Autodesk Fusion 360 part; units mm, degrees
(part 2 of 2)
  spline S180 degree 3 poles (38.6443, -77.9749) (38.4375, -77.8397) (37.9935, -77.5493) (37.4619, -77.524) (37.1779, -77.5104) knots 0 0 0 0 0.0728 0.156317 0.156317 0.156317 0.156317
  spline S181 degree 3 poles (37.1779, -77.5104) (36.8852, -77.5181) (36.3595, -77.5319) (35.9103, -77.8002) (35.7111, -77.9191) knots 0 0 0 0 0.086047 0.154532 0.154532 0.154532 0.154532
  spline S182 degree 3 poles (35.7111, -77.9191) (35.5659, -78.0588) (35.2884, -78.3257) (35.2372, -78.7061) (35.2128, -78.8875) knots 0 0 0 0 0.058494 0.11181 0.11181 0.11181 0.11181
  spline S183 degree 3 poles (35.2128, -78.8875) (35.2207, -79.0001) (35.236, -79.2199) (35.3624, -79.4) (35.424, -79.4879) knots 0 0 0 0 0.033166 0.064726 0.064726 0.064726 0.064726
  spline S184 degree 3 poles (35.424, -79.4879) (35.5146, -79.5723) (35.7243, -79.7676) (35.9938, -79.8678) (36.1469, -79.9247) knots 0 0 0 0 0.036813 0.085194 0.085194 0.085194 0.085194
  spline S185 degree 3 poles (36.1469, -79.9247) (36.3404, -79.9828) (36.8751, -80.1434) (37.4173, -80.2768) (37.7633, -80.3619) knots 0 0 0 0 0.060601 0.167477 0.167477 0.167477 0.167477
  spline S186 degree 3 poles (37.7633, -80.3619) (38.237, -80.4825) (39.0523, -80.6899) (39.7493, -81.1565) (40.0412, -81.352) knots 0 0 0 0 0.14523 0.24996 0.24996 0.24996 0.24996
  spline S187 degree 3 poles (40.0412, -81.352) (40.3097, -81.6399) (40.8404, -82.2091) (40.9213, -82.9825) (40.9613, -83.3646) knots 0 0 0 0 0.1147 0.226743 0.226743 0.226743 0.226743
  spline S188 degree 3 poles (40.9613, -83.3646) (40.9427, -83.6159) (40.9051, -84.1229) (40.6564, -84.5664) (40.531, -84.7901) knots 0 0 0 0 0.074618 0.150525 0.150525 0.150525 0.150525
  spline S189 degree 3 poles (40.531, -84.7901) (40.3663, -85.001) (40.0277, -85.4343) (39.5352, -85.6799) (39.2822, -85.806) knots 0 0 0 0 0.07921 0.162795 0.162795 0.162795 0.162795
  spline S190 degree 3 poles (39.2822, -85.806) (38.9841, -85.9072) (38.3455, -86.124) (37.6706, -86.1429) (37.3108, -86.153) knots 0 0 0 0 0.093909 0.201185 0.201185 0.201185 0.201185
  spline S191 degree 3 poles (37.3108, -86.153) (36.7447, -86.1362) (35.7243, -86.1059) (34.8636, -85.5666) (34.4803, -85.3265) knots 0 0 0 0 0.16619 0.299601 0.299601 0.299601 0.299601
  spline S192 degree 3 poles (34.4803, -85.3265) (34.1997, -85.0227) (33.6242, -84.3996) (33.5278, -83.5554) (33.4784, -83.1228) knots 0 0 0 0 0.120771 0.247752 0.247752 0.247752 0.247752
  line L111 (33.4784, -83.1228) -> (35.4976, -83.035)
  spline S193 degree 3 poles (35.4976, -83.035) (35.5448, -83.2666) (35.6308, -83.6881) (35.9243, -83.9998) (36.0565, -84.1402) knots 0 0 0 0 0.069259 0.12604 0.12604 0.12604 0.12604
  spline S194 degree 3 poles (36.0565, -84.1402) (36.2292, -84.2394) (36.622, -84.4649) (37.077, -84.4758) (37.3319, -84.4818) knots 0 0 0 0 0.058882 0.13389 0.13389 0.13389 0.13389
  spline S195 degree 3 poles (37.3319, -84.4818) (37.5994, -84.4735) (38.088, -84.4583) (38.5162, -84.226) (38.71, -84.1209) knots 0 0 0 0 0.078964 0.14421 0.14421 0.14421 0.14421
  spline S196 degree 3 poles (38.71, -84.1209) (38.8035, -84.0374) (38.9896, -83.8713) (39.0171, -83.6235) (39.0308, -83.5003) knots 0 0 0 0 0.03624 0.072106 0.072106 0.072106 0.072106
  spline S197 degree 3 poles (39.0308, -83.5003) (39.017, -83.3851) (38.9885, -83.148) (38.8184, -82.9797) (38.7309, -82.893) knots 0 0 0 0 0.033757 0.069526 0.069526 0.069526 0.069526
  spline S198 degree 3 poles (38.7309, -82.893) (38.5157, -82.776) (37.9337, -82.4593) (37.2848, -82.3148) (36.8758, -82.2238) knots 0 0 0 0 0.073213 0.198019 0.198019 0.198019 0.198019
  spline S199 degree 3 poles (36.8758, -82.2238) (36.444, -82.1199) (35.6975, -81.9404) (34.9958, -81.6305) (34.7001, -81.4998) knots 0 0 0 0 0.132891 0.229702 0.229702 0.229702 0.229702
  spline S200 degree 3 poles (34.7001, -81.4998) (34.4777, -81.3668) (34.0388, -81.1043) (33.7419, -80.6882) (33.5955, -80.483) knots 0 0 0 0 0.076824 0.151588 0.151588 0.151588 0.151588
  spline S201 degree 3 poles (33.5955, -80.483) (33.4783, -80.248) (33.2292, -79.7483) (33.206, -79.1895) (33.1937, -78.8935) knots 0 0 0 0 0.077881 0.165602 0.165602 0.165602 0.165602
  spline S202 degree 3 poles (33.1937, -78.8935) (33.2144, -78.6104) (33.2563, -78.0391) (33.5325, -77.5371) (33.6718, -77.2839) knots 0 0 0 0 0.084071 0.169684 0.169684 0.169684 0.169684
  spline S203 degree 3 poles (33.6718, -77.2839) (33.85, -77.0487) (34.2124, -76.5704) (34.7497, -76.3021) (35.0229, -76.1657) knots 0 0 0 0 0.087239 0.177491 0.177491 0.177491 0.177491
  spline S204 degree 3 poles (35.0229, -76.1657) (35.3472, -76.0606) (36.0537, -75.8316) (36.797, -75.8144) (37.1991, -75.8051) knots 0 0 0 0 0.101736 0.22162 0.22162 0.22162 0.22162
  spline S205 degree 3 poles (37.1991, -75.8051) (37.7745, -75.8258) (38.8261, -75.8638) (39.7108, -76.4252) (40.1114, -76.6794) knots 0 0 0 0 0.169048 0.308955 0.308955 0.308955 0.308955
  spline S206 degree 3 poles (40.1114, -76.6794) (40.4175, -77.0219) (41.0709, -77.7529) (41.2365, -78.7225) (41.3245, -79.2379) knots 0 0 0 0 0.135061 0.288292 0.288292 0.288292 0.288292
  line L112 (52.4787, -75.9887) -> (52.4757, -83.2329)
  line L113 (52.4757, -83.2329) -> (50.5589, -83.2322)
  line L114 (50.5589, -83.2322) -> (50.5619, -75.988)
  line L115 (50.5619, -75.988) -> (52.4787, -75.9887)
  line L116 (61.1896, -75.5148) -> (59.0001, -75.2479)
  spline S207 degree 3 poles (59.0001, -75.2479) (58.9811, -75.1348) (58.9475, -74.9339) (58.8086, -74.7868) (58.7479, -74.7226) knots 0 0 0 0 0.033474 0.059441 0.059441 0.059441 0.059441
  spline S208 degree 3 poles (58.7479, -74.7226) (58.633, -74.6631) (58.365, -74.5245) (58.0618, -74.5201) (57.8885, -74.5176) knots 0 0 0 0 0.038336 0.089411 0.089411 0.089411 0.089411
  spline S209 degree 3 poles (57.8885, -74.5176) (57.6662, -74.5204) (57.2757, -74.5254) (56.9173, -74.6769) (56.7629, -74.7422) knots 0 0 0 0 0.065896 0.115738 0.115738 0.115738 0.115738
  spline S210 degree 3 poles (56.7629, -74.7422) (56.6829, -74.8026) (56.5136, -74.9303) (56.4266, -75.1242) (56.3807, -75.2264) knots 0 0 0 0 0.029599 0.062576 0.062576 0.062576 0.062576
  spline S211 degree 3 poles (56.3807, -75.2264) (56.3551, -75.3391) (56.2894, -75.6281) (56.2908, -75.9251) (56.2917, -76.1063) knots 0 0 0 0 0.034582 0.088686 0.088686 0.088686 0.088686
  line L117 (56.2917, -76.1063) -> (56.2913, -77.1636)
  spline S212 degree 3 poles (56.2913, -77.1636) (56.5895, -76.8216) (57.1681, -76.1581) (58.039, -76.0457) (58.4609, -75.9912) knots 0 0 0 0 0.131116 0.254371 0.254371 0.254371 0.254371
  spline S213 degree 3 poles (58.4609, -75.9912) (58.9233, -76.0445) (59.8558, -76.152) (60.4655, -76.8666) (60.7728, -77.2268) knots 0 0 0 0 0.134391 0.271005 0.271005 0.271005 0.271005
  spline S214 degree 3 poles (60.7728, -77.2268) (60.9675, -77.5839) (61.3794, -78.3397) (61.4193, -79.2011) (61.4403, -79.6555) knots 0 0 0 0 0.120415 0.254815 0.254815 0.254815 0.254815
  spline S215 degree 3 poles (61.4403, -79.6555) (61.4192, -80.2082) (61.3806, -81.2201) (60.8203, -82.058) (60.566, -82.4382) knots 0 0 0 0 0.162117 0.296779 0.296779 0.296779 0.296779
  spline S216 degree 3 poles (60.566, -82.4382) (60.255, -82.7186) (59.6331, -83.2793) (58.7995, -83.3592) (58.3828, -83.3991) knots 0 0 0 0 0.122143 0.244248 0.244248 0.244248 0.244248
  spline S217 degree 3 poles (58.3828, -83.3991) (57.951, -83.3448) (57.0641, -83.2334) (56.4708, -82.5623) (56.1664, -82.2181) knots 0 0 0 0 0.126112 0.258965 0.258965 0.258965 0.258965
  line L118 (56.1664, -82.2181) -> (56.166, -83.2345)
  line L119 (56.166, -83.2345) -> (54.372, -83.2337)
  line L120 (54.372, -83.2337) -> (54.3747, -76.733)
  spline S218 degree 3 poles (54.3747, -76.733) (54.3764, -76.3576) (54.3793, -75.7104) (54.5255, -75.0808) (54.5869, -74.8163) knots 0 0 0 0 0.112164 0.193367 0.193367 0.193367 0.193367
  spline S219 degree 3 poles (54.5869, -74.8163) (54.6601, -74.6206) (54.798, -74.2523) (55.0586, -73.9584) (55.1808, -73.8207) knots 0 0 0 0 0.062057 0.116815 0.116815 0.116815 0.116815
  spline S220 degree 3 poles (55.1808, -73.8207) (55.325, -73.7049) (55.6332, -73.4576) (56.0059, -73.3253) (56.2042, -73.2549) knots 0 0 0 0 0.055092 0.117678 0.117678 0.117678 0.117678
  spline S221 degree 3 poles (56.2042, -73.2549) (56.443, -73.1955) (56.9711, -73.064) (57.5157, -73.0556) (57.8141, -73.051) knots 0 0 0 0 0.073583 0.162748 0.162748 0.162748 0.162748
  spline S222 degree 3 poles (57.8141, -73.051) (58.3519, -73.0556) (59.2781, -73.0637) (60.0871, -73.5024) (60.4264, -73.6864) knots 0 0 0 0 0.158198 0.272432 0.272432 0.272432 0.272432
  spline S223 degree 3 poles (60.4264, -73.6864) (60.6511, -73.9087) (61.0972, -74.3499) (61.1636, -74.9735) (61.1965, -75.2829) knots 0 0 0 0 0.091778 0.182191 0.182191 0.182191 0.182191
  spline S224 degree 3 poles (61.1965, -75.2829) (61.1962, -75.3182) (61.1953, -75.3955) (61.1916, -75.4728) (61.1896, -75.5148) knots 0 0 0 0 0.010574 0.023204 0.023204 0.023204 0.023204
  line L121 (119.8835, -31.5825) -> (97.8835, -31.5825)
  line L122 (97.8835, -31.5825) -> (97.8835, 28.4175)
  line L123 (97.8835, 28.4175) -> (119.8835, 28.4175)
  line L124 (119.8835, 28.4175) -> (119.8835, -31.5825)
  line L125 (119.8835, -31.5825) -> (97.8835, 28.4175) construction
  line L126 (97.8835, -31.5825) -> (119.8835, 28.4175) construction
  point P0 (108.8835, -1.5825)
  dimension "d74" = 60
  dimension "d75" = 22
  constraint horizontal L121
  constraint perpendicular L121 L122
  constraint parallel L121 L123
  constraint parallel L122 L124
  constraint coincident L125 P0
  constraint coincident L126 P0
  measures "d74" distance of L121.end L122.end
  measures "d75" distance of L121.start L121.end
extrude "Extrusion13" cut sketch "Esquisse11" against normal blind 2 contours L121 L122 L123 L124 bodies 2
extrude "Extrusion11" [suppressed]
shell "Coque4" [suppressed]
named bodies: "bas", "haut", "support carte", "support capteur gauche", "support capteur droit", "bouton gauche", "bouton droit"
